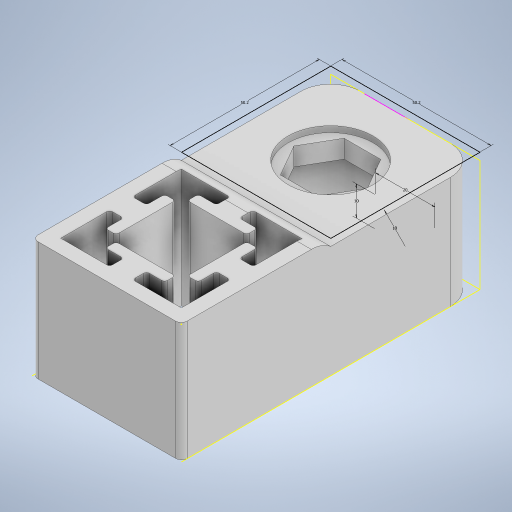
# Autodesk Inventor part: 프로파일끼울거1ver0.3
Saved by Autodesk Inventor 2023 (Build 270158000, 158)
## iProperties
Created: 2023-10-31
Part Number: 프로파일끼울거1ver0.3
Material: 일반
Document SubType Name: Modeling
Designer: rlatk
Density: 1 g/cm^3
Appearance: 기본값
Author: rlatk
Autodesk Inventor part; units mm, degrees
ref_plane "YZ Plane" through (0, 0, 0) normal (1, 0, 0) x (0, 1, 0)
ref_plane "XZ Plane" through (0, 0, 0) normal (0, 1, 0) x (-1, 0, 0)
ref_plane "XY Plane" through (0, 0, 0) normal (0, 0, 1) x (1, 0, 0)
sketch "스케치1" plane through (0, 0, 0) normal (0, 1, 0) x (-1, 0, 0)
  line L0 (0, 0) -> (50.2, 0)
  line L1 (50.2, 0) -> (50.2, -50.2)
  line L2 (50.2, -50.2) -> (0, -50.2)
  line L3 (0, -50.2) -> (0, 0)
  line L4 (45.4, -45.4) -> (4.8, -45.4)
  line L5 (4.8, -45.4) -> (4.8, -4.8)
  line L6 (4.8, -4.8) -> (45.4, -4.8)
  line L7 (45.4, -4.8) -> (45.4, -45.4)
  line L8 (28.95, -45.4) -> (21.25, -45.4)
  line L9 (21.25, -45.4) -> (21.25, -40.7)
  line L10 (21.25, -40.7) -> (28.95, -40.7)
  line L11 (28.95, -40.7) -> (28.95, -45.4)
  line L12 (35.05, -40.7) -> (15.15, -40.7)
  line L13 (15.15, -40.7) -> (15.15, -37.1)
  line L14 (15.15, -37.1) -> (35.05, -37.1)
  line L15 (35.05, -37.1) -> (35.05, -40.7)
  line L16 (40.7, -15.15) -> (40.7, -35.05)
  line L17 (37.1, -15.15) -> (40.7, -15.15)
  line L18 (37.1, -35.05) -> (37.1, -15.15)
  line L19 (40.7, -35.05) -> (37.1, -35.05)
  line L20 (45.4, -28.95) -> (40.7, -28.95)
  line L21 (40.7, -21.25) -> (45.4, -21.25)
  line L22 (15.15, -9.5) -> (35.05, -9.5)
  line L23 (15.15, -13.1) -> (15.15, -9.5)
  line L24 (35.05, -13.1) -> (15.15, -13.1)
  line L25 (35.05, -9.5) -> (35.05, -13.1)
  line L26 (28.95, -4.8) -> (28.95, -9.5)
  line L27 (21.25, -9.5) -> (21.25, -4.8)
  line L28 (9.5, -35.05) -> (9.5, -15.15)
  line L29 (13.1, -35.05) -> (9.5, -35.05)
  line L30 (13.1, -15.15) -> (13.1, -35.05)
  line L31 (9.5, -15.15) -> (13.1, -15.15)
  line L32 (4.8, -21.25) -> (9.5, -21.25)
  line L33 (9.5, -28.95) -> (4.8, -28.95)
  point P0 (25.1, -45.4)
  point P1 (25.1, -40.7)
  point P2 (28.95, -45.4)
  point P3 (28.95, -40.7)
  point P4 (21.25, -40.7)
  point P5 (21.25, -45.4)
  point P6 (25.1, -25.1)
  point P7 (40.7, -25.1)
  point P8 (25.1, -9.5)
  point P9 (9.5, -25.1)
  dimension "d0" = 50.2
  dimension "d1" = 50.2
  dimension "d2" = 40.6
  dimension "d3" = 40.6
  dimension "d4" = 4.8
  dimension "d5" = 4.8
  dimension "d6" = 7.7
  dimension "d7" = 4.7
  dimension "d8" = 19.9
  dimension "d9" = 3.6
  dimension "d55" = 360
  constraints: 68 end point, 8 parallel, 4 horizontal, 4 midpoint, 4 perpendicular, 61 other
  measures "d0" distance of L1.end L2.end
  measures "d1" distance of L0.end L1.end
  measures "d2" distance of L5.end L6.end
  measures "d3" distance of L4.end L5.end
  measures "d4" distance between parallel lines of L1 L7
  measures "d5" distance between parallel lines of L4 L2
  measures "d6" distance of L9.end L10.end
  measures "d7" distance of L8.end L9.end
  measures "d8" distance of L13.end L14.end
  measures "d9" distance of L12.end L13.end
extrude "돌출7" add sketch "스케치1" along normal blind 40 contours L0 L1 L2 L3 | L4 L9 L10 L11 | L20 L16 L21 L7 | L10 L12 L13 L14 L15 | L16 L19 L18 L17 | L5 L32 L28 L33 | L26 L22 L27 L6 | L28 L31 L30 L29 | L22 L25 L24 L23
fillet "모깎기4" radius 1 8 edges at (-15.15, 20, -40.7) (-15.15, 20, -37.1) (-21.25, 20, -45.4) (-21.25, 20, -40.7) (-28.95, 20, -45.4) (-28.95, 20, -40.7) (-35.05, 20, -40.7) (-35.05, 20, -37.1)
fillet "모깎기5" radius 1 24 edges at (-9.5, 20, -35.05) (-4.8, 20, -28.95) (-9.5, 20, -28.95) (-13.1, 20, -35.05) (-13.1, 20, -15.15) (-9.5, 20, -15.15) (-9.5, 20, -21.25) (-4.8, 20, -21.25) (-15.15, 20, -13.1) (-15.15, 20, -9.5) (-21.25, 20, -9.5) (-21.25, 20, -4.8) (-28.95, 20, -9.5) (-28.95, 20, -4.8) (-35.05, 20, -9.5) (-35.05, 20, -13.1) (-37.1, 20, -15.15) (-40.7, 20, -15.15) (-40.7, 20, -21.25) (-45.4, 20, -21.25) (-37.1, 20, -35.05) (-40.7, 20, -35.05) (-40.7, 20, -28.95) (-45.4, 20, -28.95)
sketch "스케치8" plane through (0, 40, 0) normal (0, 1, 0) x (1, 0, 0)
  line L0 (0, 50.2) -> (-50.2, 50.2) projected
  line L1 (0, 50.2) -> (-50.2, 50.2)
  line L2 (-50.2, 50.2) -> (-50.2, 100.4)
  line L3 (-50.2, 100.4) -> (0, 100.4)
  line L4 (0, 100.4) -> (0, 50.2)
  point P0 (0, 0)
  dimension "d61" = 50.2
  dimension "d62" = 50.2
  constraints: 8 end point, 2 parallel, 1 horizontal, 1 perpendicular
  measures "d61" distance of L2.end L3.end
  measures "d62" distance of L1.end L2.end
extrude "돌출8" add sketch "스케치8" against normal blind 40
sketch "스케치9" plane through (0, 40, 0) normal (0, 1, 0) x (1, 0, 0)
  line L0 (-50.2, 100.4) -> (0, 100.4) projected
  line L1 (-50.2, 50.2) -> (-50.2, 100.4) projected
  line L2 (0, 50.2) -> (-50.2, 50.2) projected
  line L3 (0, 0) -> (0, 100.4) projected
  line L4 (-37.4553, 75.3) -> (-31.2776, 86)
  line L5 (-31.2776, 86) -> (-18.9224, 86)
  line L6 (-18.9224, 86) -> (-12.7447, 75.3)
  line L7 (-12.7447, 75.3) -> (-18.9224, 64.6)
  line L8 (-18.9224, 64.6) -> (-31.2776, 64.6)
  line L9 (-31.2776, 64.6) -> (-37.4553, 75.3)
  point P0 (-25.1, 75.3)
  point P1 (-25.1, 75.3)
  dimension "d65" = 21.4
  constraints: 12 end point, 1 coincident, 13 other
  measures "d65" distance between parallel lines of L8 L5
extrude "돌출9" cut sketch "스케치9" against normal blind 40 contours L4 L5 L6 L7 L8 L9
extrude "돌출10" cut sketch "스케치8" against normal blind 2.4
sketch "스케치10" plane through (0, 37.6, 0) normal (0, 1, 0) x (1, 0, 0)
  line L0 (-50.2, 100.4) -> (0, 100.4) projected
  line L1 (-50.2, 50.2) -> (-50.2, 100.4) projected
  line L2 (0, 50.2) -> (-50.2, 50.2) projected
  line L3 (0, 100.4) -> (0, 50.2) projected
  line L4 (-18.9224, 64.6) -> (-12.7447, 75.3) projected
  line L5 (-31.2776, 64.6) -> (-18.9224, 64.6) projected
  line L6 (-37.4553, 75.3) -> (-31.2776, 64.6) projected
  line L7 (-31.2776, 86) -> (-37.4553, 75.3) projected
  line L8 (-18.9224, 86) -> (-31.2776, 86) projected
  line L9 (-12.7447, 75.3) -> (-18.9224, 86) projected
  line L10 (-50.2, 100.4) -> (0, 100.4) projected
  line L11 (-50.2, 50.2) -> (-50.2, 100.4) projected
  line L12 (0, 50.2) -> (-50.2, 50.2) projected
  line L13 (0, 100.4) -> (0, 50.2) projected
  circle A0 centre (-25.1, 75.3) radius 14.25
  point P0 (0, 0)
  point P1 (-25.1, 75.3)
  dimension "d87" = 28.5
  constraints: 1 centre point
  measures "d87" diameter of A0
sketch "스케치11" plane through (0, 0, 0) normal (0, -1, 0) x (1, 0, 0)
  line L0 (0, -50.2) -> (-50.2, -50.2) projected
  line L1 (0, 0) -> (0, -100.4) projected
  line L2 (-50.2, -100.4) -> (0, -100.4) projected
  line L3 (-50.2, 0) -> (-50.2, -100.4) projected
sketch "스케치12" plane through (0, 0, -100.4) normal (0, 0, -1) x (-1, 0, 0)
  line L0 (0, 37.6) -> (0, 0) projected
  line L1 (11.35, 37.6) -> (38.85, 37.6) projected
  line L2 (0, 40) -> (50.2, 40) projected
  line L3 (50.2, 37.6) -> (0, 37.6) projected
  line L4 (0, 37.6) -> (0, 0) projected
  line L5 (50.2, 0) -> (0, 0) projected
  line L6 (50.2, 37.6) -> (50.2, 0) projected
  line L7 (15.1, 0) -> (35.1, 0)
  line L8 (35.1, 0) -> (35.1, 10)
  line L9 (35.1, 10) -> (15.1, 10)
  line L10 (15.1, 10) -> (15.1, 0)
  arc A0 (35.1, 0) -> (25.1, 10) centre (25.1, 0) ccw
  point P0 (25.1, 0)
  dimension "d76" = 20
  dimension "d77" = 10
  dimension "d78" = 10
  constraints: 8 end point, 3 midpoint, 2 parallel, 2 point on circle, 1 centre point, 1 horizontal, 1 perpendicular, 1 point on line
  measures "d76" distance of L9.end L8.end
  measures "d77" distance of L8.end L7.end
  measures "d78" radius of A0
sketch "스케치13" plane through (0, 0, 0) normal (0, -1, 0) x (1, 0, 0)
  line L0 (-50.2, -100.4) -> (0, -100.4) projected
  circle A0 centre (-25.1, -75.3) radius 13.75 projected
  circle A1 centre (-25.1, -75.3) radius 15.5
  point P0 (0, 0)
  dimension "d84" = 31
  constraints: 1 centre point, 1 coincident
  measures "d84" diameter of A1
extrude "돌출13" cut sketch "스케치12" against normal blind 8.4 contours L10 L9 A0 L5
fillet "모깎기6" radius 10 3 edges at (-50.2, 18.8, -100.4) (0, 18.8, -100.4) (-25.1, 40, -50.2)
fillet "모깎기7" radius 2 2 edges at (0, 20, 0) (-50.2, 20, 0)
extrude "돌출14" cut sketch "스케치13" against normal blind 19.5 contours A0 | A1
extrude "돌출15" cut sketch "스케치10" against normal blind 12 contours L5 L6 L7 L8 L9 L4 | A0
sketch "스케치14" plane through (0, 0, -92) normal (0, 0, -1) x (-1, 0, 0)
  point P0 (0, 0)
sketch "스케치15" plane through (0, 0, -92) normal (0, 0, -1) x (-1, 0, 0)
  point P0 (0, 0)
sketch "스케치16" plane through (0, 0, -92) normal (0, 0, -1) x (-1, 0, 0)
  line L0 (15.1, 10) -> (25.1, 10) projected
  line L1 (15.1, 0) -> (15.1, 10) projected
  line L2 (35.1, 0) -> (15.1, 0) projected
  arc A0 (35.1, 0) -> (25.1, 10) centre (25.1, 0) ccw projected
  circle A1 centre (25.1, 0) radius 10
  line L3 (15.1, 0) -> (35.1, 0)
  line L4 (45.4, 0) -> (29.95, 0) projected
  point P0 (0, 0)
  constraints: 2 end point, 1 coincident, 1 collinear, 3 other
extrude "돌출16" cut sketch "스케치16" against normal blind 10 contours A0 L2 A1
sketch "스케치17" plane through (-25.1, 25.6, -75.3) normal (0, 1, 0) x (1, 0, 0)
  line L0 (6.1776, -10.7) -> (12.3553, 0) projected
  line L1 (-6.1776, -10.7) -> (6.1776, -10.7) projected
  line L2 (-12.3553, 0) -> (-6.1776, -10.7) projected
  line L3 (-6.1776, 10.7) -> (-12.3553, 0) projected
  line L4 (6.1776, 10.7) -> (-6.1776, 10.7) projected
  line L5 (12.3553, 0) -> (6.1776, 10.7) projected
  circle A0 centre (0, 0) radius 14.25 projected
  point P0 (25.1, -75.3)
extrude "돌출17" add sketch "스케치17" along normal blind 10
sketch "스케치18" plane through (-25.1, 19.5, -75.3) normal (0, -1, 0) x (1, 0, 0)
  line L0 (-12.3553, 0) -> (-6.1776, -10.7) projected
  line L1 (-6.1776, 10.7) -> (-12.3553, 0) projected
  line L2 (6.1776, 10.7) -> (-6.1776, 10.7) projected
  line L3 (12.3553, 0) -> (6.1776, 10.7) projected
  line L4 (6.1776, -10.7) -> (12.3553, 0) projected
  line L5 (-6.1776, -10.7) -> (6.1776, -10.7) projected
  circle A0 centre (0, 0) radius 15.5 projected
  point P0 (25.1, 75.3)
extrude "돌출18" cut sketch "스케치18" against normal blind 10
extrude "돌출19" cut sketch "스케치12" against normal blind 8.4 contours A0 L9 L8
sketch "스케치19" plane through (-15.1, 0, -100.4) normal (0, 0, -1) x (-1, 0, 0)
  line L0 (20, 10) -> (0, 10) projected
  line L1 (0, 10) -> (0, 0) projected
  line L2 (20, 0) -> (20, 10) projected
  line L3 (0, 10) -> (20, 10)
  line L4 (20, 10) -> (20, 15)
  line L5 (20, 15) -> (0, 15)
  line L6 (0, 15) -> (0, 10)
  point P0 (-15.1, 0)
  point P1 (20, 10)
  dimension "d98" = 20
  dimension "d99" = 5
  constraints: 8 end point, 2 parallel, 1 horizontal, 1 perpendicular
  measures "d98" distance of L5.end L4.end
  measures "d99" distance of L4.end L3.end
extrude "돌출20" cut sketch "스케치19" against normal blind 8.4
sketch "스케치20" plane through (0, 0, -92) normal (0, 0, -1) x (-1, 0, 0)
  arc A0 (35.1, 0) -> (15.1, 0) centre (25.1, 0) ccw projected
  line L0 (35.1, 15) -> (35.1, 0) projected
  line L1 (15.1, 15) -> (35.1, 15) projected
  line L2 (15.1, 0) -> (15.1, 15) projected
  line L3 (35.05, 0) -> (35.05, 40) projected
  arc A1 (35.05, 0) -> (22.4322, 15) centre (21.0905, 1.0644) ccw
  line L4 (22.4322, 15) -> (35.1, 15)
  line L5 (35.1, 15) -> (35.05, 0)
  point P0 (0, 0)
  point P1 (35.0568, 2.0358)
  dimension "d102" = 14
  constraints: 4 end point, 2 point on circle, 1 centre point, 1 collinear, 1 point on line
  measures "d102" radius of A1
extrude "돌출21" add sketch "스케치20" along normal blind 8.4 contours L5 A1 L3 L1 | L3 A1 L1
